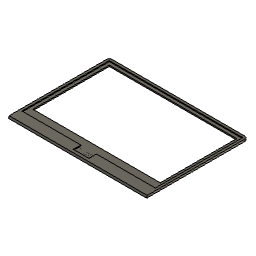
front (Autodesk Fusion 360 design; units mm, degrees)
Autodesk Fusion 360 part; units mm, degrees
sketch "Sketch1" plane through (0, 0, 0) normal (0, 0, 1) x (1, 0, 0)
  line L0 (78.2063, 84.3769) -> (241.4063, 84.3769)
  line L1 (241.4063, 84.3769) -> (241.4063, -13.5431)
  line L2 (241.4063, -13.5431) -> (78.2063, -13.5431)
  line L3 (78.2063, -13.5431) -> (78.2063, 84.3769)
  line L4 (74.7063, 87.8669) -> (244.9063, 87.8669)
  line L5 (244.9063, 87.8669) -> (244.9063, -23.3331)
  line L6 (244.9063, -23.3331) -> (74.7063, -23.3331)
  line L7 (74.7063, -23.3331) -> (74.7063, 87.8669)
  line L8 (74.7063, 87.8669) -> (244.9063, 87.8669)
  line L9 (244.9063, 87.8669) -> (244.9063, -33.3331)
  line L10 (244.9063, -33.3331) -> (74.7063, -33.3331)
  line L11 (74.7063, -33.3331) -> (74.7063, 87.8669)
  line L12 (149.8063, -33.3331) -> (169.8063, -33.3331)
  line L13 (169.8063, -33.3331) -> (169.8063, -23.3331)
  line L14 (169.8063, -23.3331) -> (149.8063, -23.3331)
  line L15 (149.8063, -23.3331) -> (149.8063, -33.3331)
  line L16 (71.3063, 91.2669) -> (248.3063, 91.2669)
  line L17 (248.3063, 91.2669) -> (248.3063, -36.7331)
  line L18 (248.3063, -36.7331) -> (71.3063, -36.7331)
  line L19 (71.3063, -36.7331) -> (71.3063, 91.2669)
  line L20 (74.3063, 88.2669) -> (245.3063, 88.2669)
  line L21 (245.3063, 88.2669) -> (245.3063, -23.7331)
  line L22 (245.3063, -23.7331) -> (74.3063, -23.7331)
  line L23 (74.3063, -23.7331) -> (74.3063, 88.2669)
  dimension "d1" = 97.92
  dimension "d2" = 163.2
  dimension "d3" = 170.2
  dimension "d4" = 3.5
  dimension "d5" = 111.2
  dimension "d6" = 3.49
  dimension "d7" = 10
  dimension "d8" = 20
  dimension "d9" = 75.1
  dimension "d11" = -3.4
  dimension "d34" = -0.4
  dimension "d35" = 75.1
  constraint horizontal L0
  constraint vertical L1
  constraint horizontal L2
  constraint vertical L3
  constraint horizontal L4
  constraint vertical L5
  constraint horizontal L6
  constraint vertical L7
  constraint horizontal L8
  constraint vertical L9
  constraint horizontal L10
  constraint vertical L11
  constraint horizontal L12
  constraint vertical L13
  constraint horizontal L14
  constraint vertical L15
  constraint coincident L6 L13.end
  constraint coincident L10 L12.start
  measures "d1" distance of L0.start L2.end
  measures "d2" distance of L0.start L0.end
  measures "d3" distance of L4.start L4.end
  measures "d4" distance of L3 L7
  measures "d5" distance of L4.start L6.end
  measures "d6" distance of L0 L4
  measures "d7" distance of L6 L10
  measures "d8" distance of L12.start L12.end
  measures "d9" distance of L11 L15
  measures "d35" distance of L9 L13
extrude "Extrude1" add sketch "Sketch1" against normal blind 1.5 contours L4 L5 L7 L8 L9 L11 L20 L21 L22 L23 | L4 L5 L6 L7 L8 L9 L11 L14 | L6 L11 L15 L22 | L6 L9 L13 L22 | L6 L13 L14 L15 L22 | L10 L11 L15 L22 | L9 L10 L13 L22 | L10 L12 L13 L15 L22 | L16 L17 L18 L19
extrude "Extrude2" add sketch "Sketch1" along normal blind 1.2 contours L10 L11 L15 L22 | L9 L10 L13 L22 | L16 L17 L18 L19
sketch "Sketch2" plane through (71.3063, 0, 0) normal (-1, 0, 0) x (0, -1, 0)
  line L0 (-91.2669, 1.2) -> (-91.2669, -1.5)
  line L1 (-91.2669, -1.5) -> (36.7331, -1.5)
  line L2 (36.7331, -1.5) -> (36.7331, 1.2)
  line L3 (36.7331, 1.2) -> (-91.2669, 1.2)
  line L4 (36.7331, -1.5) -> (33.0912, -1.5)
  line L5 (33.0912, -1.5) -> (33.0912, 2.7)
  line L6 (33.0912, 2.7) -> (36.7331, 2.7)
  line L7 (36.7331, 2.7) -> (36.7331, -1.5)
  line L8 (36.7331, 2.7) -> (38.5941, -4.2455)
  line L9 (36.7331, 2.7) -> (43.6271, 2.7) construction
  line L10 (36.7331, -1.5) -> (39.5381, -1.5)
  line L11 (35.2766, 1.2) -> (42.4884, 1.2)
  dimension "d16" = 1.5
  dimension "d17" = 75
  constraint horizontal L4
  constraint vertical L5
  constraint horizontal L6
  constraint vertical L7
  constraint coincident L1.end L2.start
  constraint horizontal L9
  constraint perpendicular L7 L10
  constraint coincident L3 L11.start
  constraint perpendicular L7 L11
  measures "d16" distance of L3 L6
  measures "d17" angle of L8 L9
extrude "Extrude3" add sketch "Sketch2" against normal up to surface (177 mm away) contours L2 L7 L8 L10 L11
fillet "Fillet1" radius 3 2 edges at (71.3063, 91.2669, -0.15) (248.3063, 91.2669, -0.15)
sketch "Sketch3" plane through (0, 0, -1.5) normal (0, 0, -1) x (1, 0, 0)
  arc A0 (245.3063, -91.2669) -> (248.3063, -88.2669) centre (245.3063, -88.2669) ccw
  line L0 (248.3063, -88.2669) -> (248.3063, 37.8584)
  line L1 (248.3063, 37.8584) -> (71.3063, 37.8584)
  line L2 (71.3063, 37.8584) -> (71.3063, -88.2669)
  arc A1 (71.3063, -88.2669) -> (74.3063, -91.2669) centre (74.3063, -88.2669) ccw
  line L3 (74.3063, -91.2669) -> (245.3063, -91.2669)
  line L4 (78.2063, 13.5431) -> (241.4063, 13.5431)
  line L5 (241.4063, 13.5431) -> (241.4063, -84.3769)
  line L6 (241.4063, -84.3769) -> (78.2063, -84.3769)
  line L7 (78.2063, -84.3769) -> (78.2063, 13.5431)
  spline S0 degree 5 poles (168.3063, 26.3081) (168.3195, 26.3986) (168.2582, 26.6166) (167.9024, 27.0513) (166.9216, 27.7962) (164.9941, 28.7753) (162.5706, 29.5411) (159.8951, 29.8719) (157.2258, 29.6505) (154.8107, 28.9513) (152.8718, 27.9853) (151.5916, 27.0179) (151.0968, 26.2949) (151.4435, 25.9718) (152.5955, 26.024) (154.4375, 26.2989) (156.7949, 26.5955) (159.4487, 26.7323) (162.1514, 26.6209) (164.6413, 26.3369) (166.6674, 26.0492) (167.7451, 25.9733) (168.179, 26.0739) (168.2931, 26.2177) (168.3063, 26.3081) knots 0 0 0 0 0 0 0.05 0.1 0.15 0.2 0.25 0.3 0.35 0.4 0.45 0.5 0.55 0.6 0.65 0.7 0.75 0.8 0.85 0.9 0.95 1 1 1 1 1 1
  circle A2 centre (171.9063, 22.9918) radius 1.5
  circle A3 centre (147.9063, 22.9919) radius 1.5
  point P0 (159.4063, 29.7363)
  point P1 (151.3063, 26.3081)
  point P2 (159.4063, 26.6713)
  dimension "d22" = 80
  dimension "d23" = 80
  dimension "d24" = 3
  dimension "d25" = 3
  dimension "d26" = 88.1
  dimension "d27" = 88.9
  dimension "d28" = 88.1
  dimension "d29" = 24
  dimension "d30" = 3.6
  dimension "d31" = 0.0001
  dimension "d36" = 3.4
  measures "d22" distance of L0 S0.start
  measures "d23" distance of L2 P1
  measures "d24" diameter of A2
  measures "d25" diameter of A3
  measures "d26" distance of L2 P0
  measures "d27" distance of L0 P0
  measures "d28" distance of L2 P2
  measures "d29" horizontal distance of A2.centre A3.centre
  measures "d30" distance of S0.start A2.centre
  measures "d31" vertical distance of A2.centre A3.centre
  measures "d36" horizontal distance of P1 A3.centre
sketch "Sketch4" plane through (0, 0, -1.5) normal (0, 0, -1) x (1, 0, 0)
extrude "Extrude4" cut sketch "Sketch3" against normal blind 0.5 contours S0 | A2 | A3
